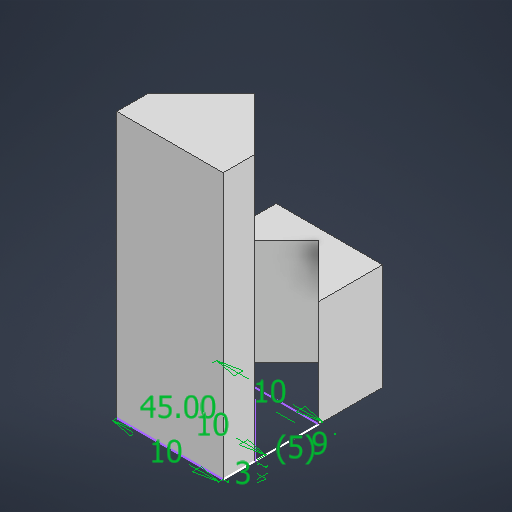
# Autodesk Inventor part: Phantom_Arm_Triangle
Saved by Autodesk Inventor 2026.2 (Build 302298000, 298)
## iProperties
Created: 2026-03-26
Part Number: Phantom_Arm_Triangle
Material: Generic
Document SubType Name: Modeling
Designer: vckot
Density: 1 g/cm^3
Appearance: Default
Author: vckot
Autodesk Inventor part; units mm, degrees
ref_plane "YZ Plane" through (0, 0, 0) normal (1, 0, 0) x (0, 1, 0)
ref_plane "XZ Plane" through (0, 0, 0) normal (0, 1, 0) x (-1, 0, 0)
ref_plane "XY Plane" through (0, 0, 0) normal (0, 0, 1) x (1, 0, 0)
sketch "Sketch1" plane through (0, 0, 0) normal (0, 0, 1) x (1, 0, 0)
  line L0 (-5, 0) -> (5, 0)
  line L1 (-5, 0) -> (0, 5)
  line L2 (-5, 0) -> (2.0711, 0) construction
  line L3 (0, 5) -> (5, 0)
  line L4 (-5, 0) -> (5, 0)
  line L5 (5, 0) -> (5, -3)
  line L6 (5, -3) -> (-5, -3)
  line L7 (-5, -3) -> (-5, 0)
  line L8 (5, -3) -> (-5, -3)
  line L9 (-5, -3) -> (-5, 6)
  line L10 (-5, 6) -> (5, 6)
  line L11 (5, 6) -> (5, -3)
  point P0 (0, 0)
  point P1 (0, 0)
  dimension "d0" = 10
  dimension "d1" = 45
  dimension "d6" = 10
  dimension "d7" = 3
  dimension "d8" = 10
  dimension "d9" = 9
  dimension "d10" = 5
  constraints: 24 end point, 4 horizontal, 4 parallel, 3 perpendicular, 1 coincident, 1 equal length, 1 midpoint
  measures "d0" distance of L0.start L0.end
  measures "d1" angle of L2 L1
  measures "d6" distance of L5.end L6.end
  measures "d7" distance of L4.end L5.end
  measures "d8" distance of L9.end L10.end
  measures "d9" distance of L10.end L5.end
  measures "d10" distance from line of L0 L1.end
extrude "Extrusion1" add sketch "Sketch1" along normal blind 25 contours L1 L3 L0 | L0 L5 L6 L7
sketch "Sketch2" plane through (0, 0, 0) normal (0, 0, -1) x (-1, 0, 0)
  line L0 (5, 6) -> (-5, 6) projected
  line L1 (-5, 6) -> (0, 11)
  line L2 (-5, 6) -> (2.0711, 6) construction
  line L3 (0, 11) -> (5, 6)
  line L4 (-5, 6) -> (-5, 12)
  line L5 (-5, 12) -> (5, 12)
  line L6 (5, 12) -> (5, 6)
  point P0 (0, 0)
  dimension "d11" = 45
  dimension "d12" = 6
  dimension "d13" = 10
  constraints: 12 end point, 2 perpendicular, 1 equal length, 1 horizontal, 1 vertical
  measures "d11" angle of L2 L1
  measures "d12" distance of L0.end L4.end
  measures "d13" distance of L4.end L5.end
extrude "Extrusion2" add sketch "Sketch2" against normal blind 10 separate body contours L3 L1 L4 L5 L6
body "Solid1"
body "Solid2"
